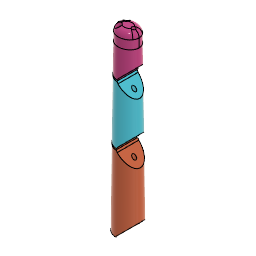
Middle Finger (Autodesk Fusion 360 design; units mm, degrees)
part number: 2025-12-07-22-56-40-952
part number: 2025-12-07-22-56-49-577
part number: 2025-12-07-23-02-24-019
part number: 2025-12-07-23-08-42-847
Autodesk Fusion 360 part; units mm, degrees
note: some values were not read from the file. Set by a fixed rule: which sketch regions a step uses.
sketch "Sketch1" plane through (0, 0, 0) normal (0, 0, 1) x (1, 0, 0) in component "Proximal phalanx"
  ellipse E0 centre (0, 0) end of major axis (0, -8) minor radius 9
  line L0 (0, 8) -> (0, -8) construction
  line L1 (-9, 0) -> (9, 0) construction
  dimension "d1" = 16
  dimension "d2" = 18
  constraint coincident E0 L0.start
  constraint coincident E0 L0.end
  constraint coincident E0 L1.start
  constraint coincident E0 L1.end
  constraint coincident E0.centre origin
  constraint vertical L0
  measures "d1" distance of E0
ref_plane "WorkPlane1" through (0, 0, 52) normal (0, 0, 1) x (1, 0, 0) in component "Proximal phalanx"
sketch "Sketch2" plane through (0, 0, 52) normal (0, 0, 1) x (1, 0, 0) in component "Proximal phalanx"
  ellipse E0 centre (0, 0) end of major axis (9, 0) minor radius 8
  spline S0 degree 3 poles (-8.5, 0) (-8.5, -1.9809) (-7.5678, -3.9555) (-5.9496, -5.3552) (-4.3409, -6.7467) (-2.0718, -7.5435) (0.1929, -7.4981) (2.4418, -7.453) (4.6517, -6.5789) (6.1851, -5.1433) (7.7507, -3.6775) (8.5942, -1.6537) (8.4912, 0.3409) (8.3892, 2.3178) (7.3573, 4.2529) (5.67, 5.5864) (4, 6.9062) (1.7075, 7.6114) (-0.5409, 7.4848) (-2.8117, 7.3569) (-5.0016, 6.3824) (-6.4678, 4.8651) (-7.7718, 3.5155) (-8.5, 1.7593) (-8.5, 0) knots -3.141593 -3.141593 -3.141593 -3.141593 -2.342572 -2.342572 -2.342572 -1.548245 -1.548245 -1.548245 -0.759463 -0.759463 -0.759463 0.045846 0.045846 0.045846 0.844037 0.844037 0.844037 1.634063 1.634063 1.634063 2.431951 2.431951 2.431951 3.141593 3.141593 3.141593 3.141593
  dimension "d4" = -0.5
loft "Loft1" add profiles "Sketch2", "Sketch1" section 1 contours S0 section 2 makes body 1 in component "Proximal phalanx"
sketch "Sketch3" plane through (0, 0, 52) normal (0, 0, 1) x (-1, 0, 0) in component "Proximal phalanx"
  spline S0 degree 3 poles (8.5, 0) (8.5, 1.9809) (7.5678, 3.9555) (5.9496, 5.3552) (4.3409, 6.7467) (2.0718, 7.5435) (-0.1929, 7.4981) (-2.4418, 7.453) (-4.6517, 6.5789) (-6.1851, 5.1433) (-7.7507, 3.6775) (-8.5942, 1.6537) (-8.4912, -0.3409) (-8.3892, -2.3178) (-7.3573, -4.2529) (-5.67, -5.5864) (-4, -6.9062) (-1.7075, -7.6114) (0.5409, -7.4848) (2.8117, -7.3569) (5.0016, -6.3824) (6.4678, -4.8651) (7.7718, -3.5155) (8.5, -1.7593) (8.5, 0) knots -3.141593 -3.141593 -3.141593 -3.141593 -2.342572 -2.342572 -2.342572 -1.548245 -1.548245 -1.548245 -0.759463 -0.759463 -0.759463 0.045846 0.045846 0.045846 0.844037 0.844037 0.844037 1.634063 1.634063 1.634063 2.431951 2.431951 2.431951 3.141593 3.141593 3.141593 3.141593
  line L0 (0, 0) -> (-8.5, 0)
  circle A0 centre (-4.25, 0) radius 1.25
  dimension "d5" = 2.5
  constraint coincident L0.start origin
  constraint coincident S0 L0.end
  constraint horizontal L0
  constraint midpoint L0 A0.centre
  measures "d5" diameter of A0
extrude "Extrude1" cut sketch "Sketch3" against normal blind 63 contours L0 A0 | L0 A0 bodies 1 in component "Proximal phalanx"
ref_plane "WorkPlane2" through (0, 0, 0) normal (0, 1, 0) x (0, 0, 1) in component "Proximal phalanx"
sketch "Sketch4" plane through (0, 0, 0) normal (0, 1, 0) x (1, 0, 0) in component "Proximal phalanx"
  line L0 (0, -52) -> (0, -51)
  line L1 (0, -51) -> (10.569, -40.431)
  line L2 (10.569, -40.431) -> (10.569, -52)
  line L3 (10.569, -52) -> (0, -52)
  line L4 (0, 0) -> (0, -1)
  line L5 (0, -1) -> (12, -13)
  line L6 (12, -13) -> (12, 0)
  line L7 (12, 0) -> (0, 0)
  dimension "d9" = 45
  dimension "d10" = 1
  dimension "d11" = 45
  dimension "d12" = 1
  constraint vertical L0
  constraint parallel L0 L2
  constraint perpendicular L0 L3
  constraint coincident L4.start L7.end
  constraint vertical L4
  constraint parallel L4 L6
  constraint perpendicular L4 L7
  measures "d9" angle of L1 L3
  measures "d10" distance of L0.start L0.end
  measures "d11" angle of L5 L7
  measures "d12" distance of L4.start L4.end
extrude "Extrude2" cut sketch "Sketch4" along normal mid plane 20 bodies 1 in component "Proximal phalanx"
fillet "Fillet1" radius 1 2 edges at (0, 0, 52) (0, 0, 0) on bodies 1 in component "Proximal phalanx"
sketch "Sketch5" plane through (0, 0, 52) normal (0, 0, 1) x (-1, 0, 0) in component "Proximal phalanx"
  line L0 (1, 7.4479) -> (1, -7.4479)
  spline S0 degree 3 poles (1, -7.4479) (3.1049, -7.2277) (5.1006, -6.28) (6.4678, -4.8651) (7.7718, -3.5155) (8.5, -1.7593) (8.5, 0) knots 1.687956 1.687956 1.687956 1.687956 2.431951 2.431951 2.431951 3.141593 3.141593 3.141593 3.141593
  spline S1 degree 3 poles (8.5, 0) (8.5, 1.9809) (7.5678, 3.9555) (5.9496, 5.3552) (4.6238, 6.502) (2.8513, 7.2542) (1, 7.4479) knots -3.141593 -3.141593 -3.141593 -3.141593 -2.342572 -2.342572 -2.342572 -1.687956 -1.687956 -1.687956 -1.687956
  line L1 (1, 0) -> (8.5, 0) construction
  line L2 (4.75, 0) -> (4.75, 6.2188) construction
  line L3 (4.75, 0) -> (4.75, -6.2188) construction
  circle A0 centre (4.75, 3.1094) radius 2
  circle A1 centre (4.75, -3.1094) radius 2
  dimension "d17" = 4
  dimension "d18" = 4
  constraint midpoint L0 L1.start
  constraint coincident S0.end S1.start
  constraint midpoint L1 L2.start
  constraint coincident S1 L2.end
  constraint perpendicular L1 L2
  constraint coincident S0 L3.end
  constraint perpendicular L1 L3
  constraint midpoint L2 A0.centre
  constraint midpoint L3 A1.centre
  measures "d17" diameter of A0
  measures "d18" diameter of A1
extrude "Extrude3" cut sketch "Sketch5" against normal blind 61 contours A0 | A1 bodies 1 in component "Proximal phalanx"
ref_plane "WorkPlane1" through (-4.75, 0, 53) normal (0, 0, 1) x (1, 0, 0) in component "Middle phalanx"
sketch "Sketch1 (2)" plane through (0, 0, 53) normal (0, 0, 1) x (1, 0, 0) in component "Middle phalanx"
  spline S0 degree 3 poles (-8.5, 0) (-8.5, -1.9809) (-7.5678, -3.9555) (-5.9496, -5.3552) (-4.3409, -6.7467) (-2.0718, -7.5435) (0.1929, -7.4981) (2.4418, -7.453) (4.6517, -6.5789) (6.1851, -5.1433) (7.7507, -3.6775) (8.5942, -1.6537) (8.4912, 0.3409) (8.3892, 2.3178) (7.3573, 4.2529) (5.67, 5.5864) (4, 6.9062) (1.7075, 7.6114) (-0.5409, 7.4848) (-2.8117, 7.3569) (-5.0016, 6.3824) (-6.4678, 4.8651) (-7.7718, 3.5155) (-8.5, 1.7593) (-8.5, 0) knots -3.141593 -3.141593 -3.141593 -3.141593 -2.342572 -2.342572 -2.342572 -1.548245 -1.548245 -1.548245 -0.759463 -0.759463 -0.759463 0.045846 0.045846 0.045846 0.844037 0.844037 0.844037 1.634063 1.634063 1.634063 2.431951 2.431951 2.431951 3.141593 3.141593 3.141593 3.141593
ref_plane "WorkPlane2" through (0.0471, 0.034, 93) normal (0, 0, 1) x (1, 0, 0) in component "Middle phalanx"
sketch "Sketch2 (2)" plane through (0, 0, 93) normal (0, 0, 1) x (1, 0, 0) in component "Middle phalanx"
  spline S0 degree 3 poles (-8.5, 0) (-8.5, -1.9809) (-7.5678, -3.9555) (-5.9496, -5.3552) (-4.3409, -6.7467) (-2.0718, -7.5435) (0.1929, -7.4981) (2.4418, -7.453) (4.6517, -6.5789) (6.1851, -5.1433) (7.7507, -3.6775) (8.5942, -1.6537) (8.4912, 0.3409) (8.3892, 2.3178) (7.3573, 4.2529) (5.67, 5.5864) (4, 6.9062) (1.7075, 7.6114) (-0.5409, 7.4848) (-2.8117, 7.3569) (-5.0016, 6.3824) (-6.4678, 4.8651) (-7.7718, 3.5155) (-8.5, 1.7593) (-8.5, 0) knots -3.141593 -3.141593 -3.141593 -3.141593 -2.342572 -2.342572 -2.342572 -1.548245 -1.548245 -1.548245 -0.759463 -0.759463 -0.759463 0.045846 0.045846 0.045846 0.844037 0.844037 0.844037 1.634063 1.634063 1.634063 2.431951 2.431951 2.431951 3.141593 3.141593 3.141593 3.141593
  spline S1 degree 3 poles (-8, 0) (-8, -1.8695) (-7.1026, -3.7403) (-5.5262, -5.059) (-4.0005, -6.3351) (-1.8533, -7.0611) (0.2795, -6.9957) (2.4466, -6.9293) (4.5601, -6.0458) (5.98, -4.6471) (7.5319, -3.1183) (8.2432, -1.0137) (7.9214, 0.978) (7.6312, 2.7732) (6.5022, 4.4765) (4.809, 5.592) (3.127, 6.7001) (0.9068, 7.1983) (-1.1891, 6.9221) (-3.232, 6.6529) (-5.1321, 5.6544) (-6.3644, 4.2383) (-7.4247, 3.02) (-8, 1.5088) (-8, 0) knots -3.141593 -3.141593 -3.141593 -3.141593 -2.325825 -2.325825 -2.325825 -1.536333 -1.536333 -1.536333 -0.734109 -0.734109 -0.734109 0.142683 0.142683 0.142683 0.93297 0.93297 0.93297 1.718013 1.718013 1.718013 2.483222 2.483222 2.483222 3.141593 3.141593 3.141593 3.141593
  dimension "d23" = -0.5
loft "Loft1'" add profiles "Sketch2 (2)", "Sketch1 (2)" section 1 contours S1 section 2 separate body makes body 2 in component "Middle phalanx"
sketch "Sketch3 (2)" plane through (0, 0, 93) normal (0, 0, 1) x (-1, 0, 0) in component "Middle phalanx"
  spline S0 degree 3 poles (8, 0) (8, 1.8695) (7.1026, 3.7403) (5.5262, 5.059) (4.0005, 6.3351) (1.8533, 7.0611) (-0.2795, 6.9957) (-2.4466, 6.9293) (-4.5601, 6.0458) (-5.98, 4.6471) (-7.5319, 3.1183) (-8.2432, 1.0137) (-7.9214, -0.978) (-7.6312, -2.7732) (-6.5022, -4.4765) (-4.809, -5.592) (-3.127, -6.7001) (-0.9068, -7.1983) (1.1891, -6.9221) (3.232, -6.6529) (5.1321, -5.6544) (6.3644, -4.2383) (7.4247, -3.02) (8, -1.5088) (8, 0) knots -3.141593 -3.141593 -3.141593 -3.141593 -2.325825 -2.325825 -2.325825 -1.536333 -1.536333 -1.536333 -0.734109 -0.734109 -0.734109 0.142683 0.142683 0.142683 0.93297 0.93297 0.93297 1.718013 1.718013 1.718013 2.483222 2.483222 2.483222 3.141593 3.141593 3.141593 3.141593
  line L0 (0, 0) -> (-0.5, 0)
  line L1 (-0.5, 0) -> (-8, 0) construction
  circle A0 centre (-4.25, 0) radius 1.25
  dimension "d24" = 2.5
  constraint coincident L0.start origin
  constraint horizontal L0
  constraint coincident S0 L1.end
  constraint parallel L0 L1
  constraint midpoint L1 A0.centre
  measures "d24" diameter of A0
extrude "Extrude1'" cut sketch "Sketch3 (2)" against normal blind 42 contours A0 bodies 2 in component "Middle phalanx"
ref_plane "WorkPlane3" through (0, 0, 0) normal (0, 1, 0) x (0, 0, 1) in component "Middle phalanx"
sketch "Sketch4 (2)" plane through (0, 0, 0) normal (0, 1, 0) x (1, 0, 0) in component "Middle phalanx"
  line L0 (0, -93) -> (0, -92)
  line L1 (0, -92) -> (10.5126, -81.4874)
  line L2 (10.5126, -81.4874) -> (10.5126, -93)
  line L3 (10.5126, -93) -> (0, -93)
  line L4 (0, -53) -> (0, -54)
  line L5 (0, -54) -> (9, -63)
  line L6 (9, -63) -> (9, -53)
  line L7 (9, -53) -> (0, -53)
  dimension "d28" = 1
  dimension "d29" = 45
  dimension "d30" = 1
  dimension "d31" = 45
  constraint vertical L0
  constraint parallel L0 L2
  constraint perpendicular L0 L3
  constraint vertical L4
  constraint parallel L4 L6
  constraint perpendicular L4 L7
  measures "d28" distance of L0.start L0.end
  measures "d29" angle of L1 L3
  measures "d30" distance of L4.start L4.end
  measures "d31" angle of L5 L7
extrude "Extrude2'" cut sketch "Sketch4 (2)" along normal mid plane 20 bodies 2 in component "Middle phalanx"
fillet "Fillet1'" radius 1 2 edges at (0, 0, 93) (0, 0, 53) on bodies 2 in component "Middle phalanx"
sketch "Sketch5 (2)" plane through (0, 0, 93) normal (0, 0, 1) x (-1, 0, 0) in component "Middle phalanx"
  line L0 (1, 6.945) -> (1, -6.945)
  spline S0 degree 3 poles (1, -6.945) (1.0632, -6.938) (1.1262, -6.9304) (1.1891, -6.9221) (3.232, -6.6529) (5.1321, -5.6544) (6.3644, -4.2383) (7.4247, -3.02) (8, -1.5088) (8, 0) knots 1.69445 1.69445 1.69445 1.69445 1.718013 1.718013 1.718013 2.483222 2.483222 2.483222 3.141593 3.141593 3.141593 3.141593
  spline S1 degree 3 poles (8, 0) (8, 1.8695) (7.1026, 3.7403) (5.5262, 5.059) (4.3062, 6.0794) (2.6903, 6.7583) (1, 6.945) knots -3.141593 -3.141593 -3.141593 -3.141593 -2.325825 -2.325825 -2.325825 -1.694526 -1.694526 -1.694526 -1.694526
  line L1 (1, 0) -> (8, 0) construction
  line L2 (4.5, 0) -> (4.5, -5.7857) construction
  line L3 (4.5, 0) -> (4.5, 5.7857) construction
  circle A0 centre (4.5, -2.8929) radius 2
  circle A1 centre (4.5, 2.8929) radius 2
  dimension "d36" = 4
  constraint midpoint L0 L1.start
  constraint coincident S0.end S1.start
  constraint midpoint L1 L2.start
  constraint coincident S0 L2.end
  constraint perpendicular L1 L2
  constraint coincident S1 L3.end
  constraint perpendicular L1 L3
  constraint midpoint L2 A0.centre
  constraint symmetric L1 A0 A1
  measures "d36" diameter of A0
extrude "Extrude3'" cut sketch "Sketch5 (2)" against normal blind 40 contours A0 | A1 bodies 2 in component "Middle phalanx"
ref_plane "WorkPlane1" through (-4.5, 0, 94) normal (0, 0, 1) x (1, 0, 0) in component "Distal phalanx"
sketch "Sketch1 (3)" plane through (0, 0, 94) normal (0, 0, 1) x (1, 0, 0) in component "Distal phalanx"
  spline S0 degree 3 poles (-8, 0) (-8, -1.8695) (-7.1026, -3.7403) (-5.5262, -5.059) (-4.0005, -6.3351) (-1.8533, -7.0611) (0.2795, -6.9957) (2.4466, -6.9293) (4.5601, -6.0458) (5.98, -4.6471) (7.5319, -3.1183) (8.2432, -1.0137) (7.9214, 0.978) (7.6312, 2.7732) (6.5022, 4.4765) (4.809, 5.592) (3.127, 6.7001) (0.9068, 7.1983) (-1.1891, 6.9221) (-3.232, 6.6529) (-5.1321, 5.6544) (-6.3644, 4.2383) (-7.4247, 3.02) (-8, 1.5088) (-8, 0) knots -3.141593 -3.141593 -3.141593 -3.141593 -2.325825 -2.325825 -2.325825 -1.536333 -1.536333 -1.536333 -0.734109 -0.734109 -0.734109 0.142683 0.142683 0.142683 0.93297 0.93297 0.93297 1.718013 1.718013 1.718013 2.483222 2.483222 2.483222 3.141593 3.141593 3.141593 3.141593
ref_plane "WorkPlane2" through (0.1216, 0.0686, 114) normal (0, 0, 1) x (1, 0, 0) in component "Distal phalanx"
sketch "Sketch2 (3)" plane through (0, 0, 114) normal (0, 0, 1) x (1, 0, 0) in component "Distal phalanx"
  spline S0 degree 3 poles (-8, 0) (-8, -1.8695) (-7.1026, -3.7403) (-5.5262, -5.059) (-4.0005, -6.3351) (-1.8533, -7.0611) (0.2795, -6.9957) (2.4466, -6.9293) (4.5601, -6.0458) (5.98, -4.6471) (7.5319, -3.1183) (8.2432, -1.0137) (7.9214, 0.978) (7.6312, 2.7732) (6.5022, 4.4765) (4.809, 5.592) (3.127, 6.7001) (0.9068, 7.1983) (-1.1891, 6.9221) (-3.232, 6.6529) (-5.1321, 5.6544) (-6.3644, 4.2383) (-7.4247, 3.02) (-8, 1.5088) (-8, 0) knots -3.141593 -3.141593 -3.141593 -3.141593 -2.325825 -2.325825 -2.325825 -1.536333 -1.536333 -1.536333 -0.734109 -0.734109 -0.734109 0.142683 0.142683 0.142683 0.93297 0.93297 0.93297 1.718013 1.718013 1.718013 2.483222 2.483222 2.483222 3.141593 3.141593 3.141593 3.141593
  spline S1 degree 3 poles (-7.7, 0) (-7.7, -1.78) (-6.8461, -3.5665) (-5.3278, -4.8338) (-3.8662, -6.0538) (-1.8006, -6.7554) (0.2537, -6.6964) (2.2836, -6.638) (4.2661, -5.8388) (5.6277, -4.5692) (7.1615, -3.1391) (7.8962, -1.1552) (7.6525, 0.7419) (7.4289, 2.4828) (6.3771, 4.1617) (4.7432, 5.275) (3.1703, 6.3467) (1.0712, 6.8637) (-0.9321, 6.6506) (-2.9062, 6.4406) (-4.7639, 5.5273) (-5.9896, 4.2066) (-7.0994, 3.0109) (-7.7, 1.5031) (-7.7, 0) knots -3.141593 -3.141593 -3.141593 -3.141593 -2.324761 -2.324761 -2.324761 -1.538445 -1.538445 -1.538445 -0.761499 -0.761499 -0.761499 0.113692 0.113692 0.113692 0.916821 0.916821 0.916821 1.689941 1.689941 1.689941 2.451812 2.451812 2.451812 3.141593 3.141593 3.141593 3.141593
  dimension "d41" = -0.3
loft "Loft1''" add profiles "Sketch2 (3)", "Sketch1 (3)" section 1 contours S1 section 2 separate body makes body 3 in component "Distal phalanx"
sketch "Sketch3 (3)" plane through (0, 0, 114) normal (0, 0, 1) x (-1, 0, 0) in component "Distal phalanx"
  spline S0 degree 3 poles (7.7, 0) (7.7, 1.78) (6.8461, 3.5665) (5.3278, 4.8338) (3.8662, 6.0538) (1.8006, 6.7554) (-0.2537, 6.6964) (-2.2836, 6.638) (-4.2661, 5.8388) (-5.6277, 4.5692) (-7.1615, 3.1391) (-7.8962, 1.1552) (-7.6525, -0.7419) (-7.4289, -2.4828) (-6.3771, -4.1617) (-4.7432, -5.275) (-3.1703, -6.3467) (-1.0712, -6.8637) (0.9321, -6.6506) (2.9062, -6.4406) (4.7639, -5.5273) (5.9896, -4.2066) (7.0994, -3.0109) (7.7, -1.5031) (7.7, 0) knots -3.141593 -3.141593 -3.141593 -3.141593 -2.324761 -2.324761 -2.324761 -1.538445 -1.538445 -1.538445 -0.761499 -0.761499 -0.761499 0.113692 0.113692 0.113692 0.916821 0.916821 0.916821 1.689941 1.689941 1.689941 2.451812 2.451812 2.451812 3.141593 3.141593 3.141593 3.141593
  line L0 (0, 0) -> (-7.7, 0)
  circle A0 centre (-3.85, 0) radius 1.25
  dimension "d42" = 2.5
  constraint coincident L0.start origin
  constraint coincident S0 L0.end
  constraint horizontal L0
  constraint midpoint L0 A0.centre
  measures "d42" diameter of A0
extrude "Extrude1''" cut sketch "Sketch3 (3)" against normal blind 23 contours L0 A0 | L0 A0 bodies 3 in component "Distal phalanx"
ref_plane "WorkPlane3" through (0, 0, 0) normal (0, 1, 0) x (0, 0, 1) in component "Distal phalanx"
sketch "Sketch4 (3)" plane through (0, 0, 0) normal (0, 1, 0) x (1, 0, 0) in component "Distal phalanx"
  line L0 (0, -94) -> (0, -95)
  line L1 (0, -95) -> (9, -104)
  line L2 (9, -104) -> (9, -94)
  line L3 (9, -94) -> (0, -94)
  dimension "d46" = 1
  dimension "d47" = 45
  constraint vertical L0
  constraint parallel L0 L2
  constraint perpendicular L0 L3
  measures "d46" distance of L0.start L0.end
  measures "d47" angle of L1 L3
extrude "Extrude2''" cut sketch "Sketch4 (3)" along normal mid plane 20 bodies 3 in component "Distal phalanx"
sketch "Sketch5 (3)" plane through (0, 0, 114) normal (0, 0, 1) x (-1, 0, 0) in component "Distal phalanx"
  circle A0 centre (-3.85, 0) radius 1.25
  spline S0 degree 3 poles (7.7, 0) (7.7, 1.78) (6.8461, 3.5665) (5.3278, 4.8338) (3.8662, 6.0538) (1.8006, 6.7554) (-0.2537, 6.6964) (-2.2836, 6.638) (-4.2661, 5.8388) (-5.6277, 4.5692) (-7.1615, 3.1391) (-7.8962, 1.1552) (-7.6525, -0.7419) (-7.4289, -2.4828) (-6.3771, -4.1617) (-4.7432, -5.275) (-3.1703, -6.3467) (-1.0712, -6.8637) (0.9321, -6.6506) (2.9062, -6.4406) (4.7639, -5.5273) (5.9896, -4.2066) (7.0994, -3.0109) (7.7, -1.5031) (7.7, 0) knots -3.141593 -3.141593 -3.141593 -3.141593 -2.324761 -2.324761 -2.324761 -1.538445 -1.538445 -1.538445 -0.761499 -0.761499 -0.761499 0.113692 0.113692 0.113692 0.916821 0.916821 0.916821 1.689941 1.689941 1.689941 2.451812 2.451812 2.451812 3.141593 3.141593 3.141593 3.141593
  line L0 (0, 0) -> (7.7, 0) construction
  line L1 (3.85, 0) -> (3.85, -5.8003) construction
  line L2 (3.85, -5.8003) -> (3.85, 0) construction
  line L3 (3.85, 0) -> (3.85, 5.8003) construction
  circle A1 centre (3.85, -2.9002) radius 2
  circle A2 centre (3.85, 2.9002) radius 2
  dimension "d50" = 4
  dimension "d51" = 4
  constraint coincident L0.start origin
  constraint coincident S0.start S0.end
  constraint midpoint L0 L1.start
  constraint coincident S0 L1.end
  constraint perpendicular L0 L1
  constraint coincident S0 L3.end
  constraint perpendicular L0 L3
  constraint midpoint L1 A1.centre
  constraint midpoint L3 A2.centre
  measures "d50" diameter of A1
  measures "d51" diameter of A2
extrude "Extrude3''" cut sketch "Sketch5 (3)" against normal blind 20.5 contours A1 | A2 bodies 3 in component "Distal phalanx"
extrude "Extrude4" add 1 faces at (1.1269, -3.5312, 114) along direction (0, 0, 1) blind 10 on bodies 3 bodies 3 in component "Distal phalanx"
fillet "Fillet1''" radius 4 1 edges at (7.6983, -0.0004, 124) on bodies 3 in component "Distal phalanx"
component "Proximal phalanx" placed x (1, 0, 0) y (0, 1, 0) z (0, 0, 1) at (0, 0, 0)
component "Middle phalanx" placed x (1, 0, 0) y (0, 1, 0) z (0, 0, 1) at (0, 0, 0)
component "Distal phalanx" placed x (1, 0, 0) y (0, 1, 0) z (0, 0, 1) at (0, 0, 0)
equation "d3 = 6.7 cm - 1.5 cm"
